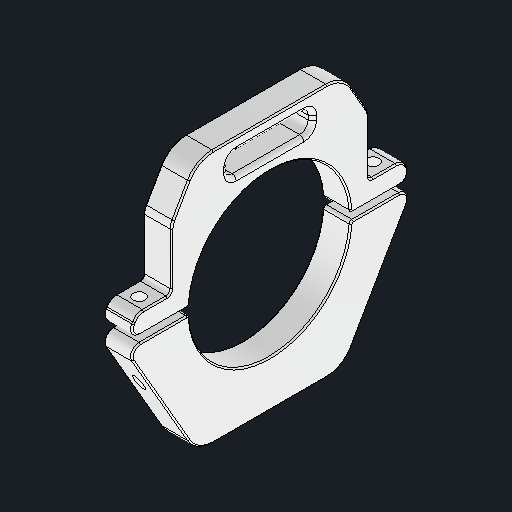
# Autodesk Inventor part: flange-camp-114
Saved by Autodesk Inventor 2027.1 (Build 311270010, 270A)
## iProperties
Created: 2026-09-25
Part Number: flange-camp-114
Material: Aluminum 6061
Document SubType Name: Modeling
Designer: queezz
Density: 2.7 g/cm^3
Appearance: Aluminum - Flat
Mass: 803.112 g
Surface Area: 567.815 cm^2
Volume: 297.449 cm^3
d0: 114,500 mm
d1: 180,000 mm
d2: 20,000 mm
d3: 0,00 deg
d4: 20,000 mm
d10: 40,000 mm
d12: 12,000 mm
d16: 30,000 mm
d17: 118,00 deg
d18: 5,000 mm
d19: 250,000 mm
d21: 0,00 deg
d22: 6,000 mm
d23: 2,000 mm
d24: 14,000 mm
d25: 70,000 mm
d26: 120,000 mm
d28: 0,00 deg
d29: 8,000 mm
d30: 10,000 mm
d31: 3,000 mm
d32: 83,000 mm
d34: 16,000 mm
d40: 8,500 mm
d46: 118,00 deg
d47: 1,000 mm
d50: 60,000 mm
d51: 15,000 mm
d53: 0,00 deg
d54: 6,000 mm
d55: 3,000 mm
hole: 114,500 mm
height: 180,000 mm
Author: queezz
Autodesk Inventor part; units mm, degrees
ref_plane "YZ Plane" through (0, 0, 0) normal (1, 0, 0) x (0, 1, 0)
ref_plane "XZ Plane" through (0, 0, 0) normal (0, 1, 0) x (-1, 0, 0)
ref_plane "XY Plane" through (0, 0, 0) normal (0, 0, 1) x (1, 0, 0)
sketch "Sketch1" plane through (0, 0, 0) normal (0, 0, 1) x (1, 0, 0)
  line L0 (51.9615, 90) -> (103.923, 0)
  line L1 (103.923, 0) -> (51.9615, -90)
  line L2 (51.9615, -90) -> (-51.9615, -90)
  line L3 (-51.9615, -90) -> (-103.923, 0)
  line L4 (-103.923, 0) -> (-51.9615, 90)
  line L5 (-51.9615, 90) -> (51.9615, 90)
  circle A0 centre (0, 0) radius 57.25
  dimension "d0" = 114.5
  dimension "d1" = 180
  constraints: 12 end point, 2 coincident, 1 centre point, 1 horizontal, 13 other
  measures "d0" diameter of A0
  measures "d1" distance between parallel lines of L2 L5
extrude "Extrusion1" add sketch "Sketch1" along normal mid plane 20
fillet "Fillet1" radius 20 4 edges at (51.9615, 90, 0) (-51.9615, 90, 0) (51.9615, -90, 0) (-51.9615, -90, 0)
sketch "M6 mounting centres - 40 mm pitch" plane through (-40.4145, 90, -9) normal (0, 1, 0) x (1, 0, 0)
  line L0 (20.4145, -9) -> (60.4145, -9) construction
  line L1 (0, 1) -> (80.829, 1) projected
  line L2 (-17.3205, 1) -> (-17.3205, -19) projected
  point P0 (40.4145, -9)
  point P1 (40.4145, -9)
  point P2 (40.4145, 1)
  point P3 (-17.3205, -9)
  point P4 (40.4145, 1)
  dimension "d18" = 5
  dimension "d19" = 250
  dimension "d54" = 6
  dimension "d10" = 40
  constraints: 4 midpoint, 2 coincident, 2 end point, 2 vertical alignment, 1 horizontal, 1 horizontal alignment
  measures "d10" distance of L0.start L0.end
hole "Hole1" at (-20, 90, 0) at (20, 90, 0) direction (0, -1, 0) diameter 4.917 depth 30 tip angle 118 thread size "M6x1" class "6H" standard "ANSI Metric M Profile"
sketch "Sketch3" plane through (0, 0, -10) normal (0, 0, -1) x (-1, 0, 0)
  line L0 (125, -2.5) -> (-125, -2.5)
  line L1 (-125, -2.5) -> (-125, 2.5)
  line L2 (-125, 2.5) -> (125, 2.5)
  line L3 (125, 2.5) -> (125, -2.5)
  point P0 (0, 0)
  point P1 (-125, 0)
  point P2 (0, -2.5)
  dimension "d18" = 5
  dimension "d19" = 250
  constraints: 8 end point, 2 midpoint, 2 parallel, 1 horizontal, 1 horizontal alignment, 1 perpendicular, 1 vertical alignment
  measures "d18" distance of L0.end L1.end
  measures "d19" distance of L0.start L0.end
extrude "Extrusion3" cut sketch "Sketch3" against normal through all
fillet "Fillet2" radius 6 4 edges at (-102.4797, -2.5, 0) (-102.4797, 2.5, 0) (102.4797, 2.5, 0) (102.4797, -2.5, 0)
fillet "Fillet3" radius 2 4 edges at (-57.1954, 2.5, 0) (-57.1954, -2.5, 0) (57.1954, 2.5, 0) (57.1954, -2.5, 0)
sketch "Sketch4" plane through (0, 0, -10) normal (0, 0, -1) x (-1, 0, 0)
  line L0 (120, -90) -> (70, -90)
  line L1 (70, -90) -> (70, -16.5)
  line L2 (70, -16.5) -> (120, -16.5)
  line L3 (120, -16.5) -> (120, -90)
  line L4 (92.0874, -2.5) -> (59.0789, -2.5) projected
  line L5 (-40.4145, -90) -> (40.4145, -90) projected
  point P0 (0, 0)
  dimension "d24" = 14
  dimension "d25" = 70
  dimension "d26" = 120
  constraints: 8 end point, 2 parallel, 1 horizontal, 1 perpendicular, 1 point on line
  measures "d24" distance between parallel lines of L4 L2
  measures "d25" distance from line of point (0, 0) L1
  measures "d26" distance from line of point (0, 0) L3
extrude "Extrusion4" cut sketch "Sketch4" against normal through all
fillet "Fillet4" radius 8 1 edges at (-94.3968, -16.5, 0)
fillet "Fillet5" radius 10 1 edges at (-70, -58.7564, 0)
fillet "Fillet6" radius 3 1 edges at (-70, -16.5, 0)
mirror "Mirror1" about plane through (0, 0, 0) normal (1, 0, 0) of "Fillet5", "Fillet4", "Extrusion4", "Fillet6"
sketch "Sketch5" plane through (-89.778, -16.5, -10) normal (0, -1, 0) x (1, 0, 0)
  line L0 (6.778, 10) -> (172.778, 10) construction
  point P0 (89.778, 10)
  point P1 (89.778, 10)
  dimension "d32" = 83
  constraints: 3 coincident, 2 end point, 1 horizontal, 1 midpoint
  measures "d32" distance of L0.start point (89.778, 10)
hole "Hole2" at (-83, -16.5, 0) at (83, -16.5, 0) direction (0, 1, 0) diameter 6.647 end through all thread size "M8x1.25" class "6H" standard "ANSI Metric M Profile"
hole "Hole3" at (-83, -16.5, 0) at (83, -16.5, 0) direction (0, 1, 0) diameter 8.5 depth 14 tip angle 118
chamfer "Chamfer2" distance 1 angle 45 72 edges at (0, -90, -10) (-50.4145, -87.3205, -10) (-63.1976, -70.5385, -10) (-69.6593, -58.6651, -10) (-70, -37.7885, -10) (-70.8787, -17.3787, -10) (-81.389, -16.5, -10) (-93.778, -15.4282, -10) (-96.9948, -12, -10) (-97.2835, -5.5, -10) (-75.5831, -2.5, -10) (-57.7194, -3.0331, -10) (0, -57.25, -10) (57.7194, -3.0331, -10) (75.5831, -2.5, -10) (97.2835, -5.5, -10) (96.9948, -12, -10) (93.778, -15.4282, -10) (81.389, -16.5, -10) (70.8787, -17.3787, -10) (70, -37.7885, -10) (69.6593, -58.6651, -10) (63.1976, -70.5385, -10) (50.4145, -87.3205, -10) (0, 57.25, 10) (57.7194, 3.0331, 10) (75.5831, 2.5, 10) (97.2835, 5.5, 10) (77.5093, 45.75, 10) (50.4145, 87.3205, 10) (0, 90, 10) (-50.4145, 87.3205, 10) (-77.5093, 45.75, 10) (-97.2835, 5.5, 10) (-75.5831, 2.5, 10) (-57.7194, 3.0331, 10) (-75.5831, 2.5, -10) (-97.2835, 5.5, -10) (-77.5093, 45.75, -10) (-50.4145, 87.3205, -10) (0, 90, -10) (50.4145, 87.3205, -10) (77.5093, 45.75, -10) (97.2835, 5.5, -10) (75.5831, 2.5, -10) (57.7194, 3.0331, -10) (0, 57.25, -10) (-57.7194, 3.0331, -10) (-70, -37.7885, 10) (-69.6593, -58.6651, 10) (-63.1976, -70.5385, 10) (-50.4145, -87.3205, 10) (0, -90, 10) (50.4145, -87.3205, 10) (63.1976, -70.5385, 10) (69.6593, -58.6651, 10) (70, -37.7885, 10) (70.8787, -17.3787, 10) (81.389, -16.5, 10) (93.778, -15.4282, 10) (96.9948, -12, 10) (97.2835, -5.5, 10) (75.5831, -2.5, 10) (57.7194, -3.0331, 10) (0, -57.25, 10) (-57.7194, -3.0331, 10) (-75.5831, -2.5, 10) (-97.2835, -5.5, 10) (-96.9948, -12, 10) (-93.778, -15.4282, 10) (-81.389, -16.5, 10) (-70.8787, -17.3787, 10)
sketch "Sketch6" plane through (0, 0, 10) normal (0, 0, 1) x (1, 0, 0)
  line L0 (30, -81.125) -> (-30, -81.125)
  line L1 (-30, -81.125) -> (-30, -66.125)
  line L2 (-30, -66.125) -> (30, -66.125)
  line L3 (30, -66.125) -> (30, -81.125)
  arc A0 (-57.0846, -4.3481) -> (57.0846, -4.3481) centre (0, 0) ccw projected
  line L4 (0, -57.25) -> (0, -90) construction
  line L5 (-40.4145, -90) -> (40.4145, -90) projected
  point P0 (0, -69.5097)
  point P1 (30, -73.625)
  point P2 (0, -73.625)
  point P3 (0, -66.125)
  dimension "d50" = 60
  dimension "d51" = 15
  constraints: 10 end point, 4 midpoint, 3 vertical alignment, 2 parallel, 1 horizontal, 1 horizontal alignment, 1 perpendicular, 1 point on circle, 1 vertical
  measures "d50" distance of L0.start L0.end
  measures "d51" distance of L0.end L1.end
extrude "Extrusion5" cut sketch "Sketch6" against normal through all
fillet "Fillet7" radius 6 4 edges at (30, -81.125, 0) (30, -66.125, 0) (-30, -81.125, 0) (-30, -66.125, 0)
fillet "Fillet8" radius 3 16 edges at (-28.2426, -79.3676, 10) (-30, -73.625, 10) (-28.2426, -67.8824, 10) (0, -66.125, 10) (28.2426, -67.8824, 10) (30, -73.625, 10) (28.2426, -79.3676, 10) (0, -81.125, 10) (28.2426, -79.3676, -10) (30, -73.625, -10) (28.2426, -67.8824, -10) (0, -66.125, -10) (-28.2426, -67.8824, -10) (-30, -73.625, -10) (-28.2426, -79.3676, -10) (0, -81.125, -10)
equation "\"d1\" = height"
equation "\"hole\" = 114.5"
equation "\"height\" = 180"
body "Solid1"
